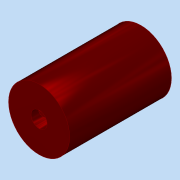
# Autodesk Inventor part: 3mm_.125inch_ShaftCoupler
Saved by Autodesk Inventor 2017.3 (Build 213256000, 256)
## iProperties
Created: 2018-07-04
Part Number: 3mm_.125inch_ShaftCoupler
Material: Aluminum 6061
Document SubType Name: Modeling
Designer: Derek Wider
Density: 2.7 g/cm^3
Appearance: Red Adonized
Author: Derek Wider
Autodesk Inventor part; units mm, degrees
ref_plane "YZ Plane" through (0, 0, 0) normal (1, 0, 0) x (0, 1, 0)
ref_plane "XZ Plane" through (0, 0, 0) normal (0, 1, 0) x (-1, 0, 0)
ref_plane "XY Plane" through (0, 0, 0) normal (0, 0, 1) x (1, 0, 0)
sketch "Sketch1" plane through (0, 0, 0) normal (0, 0, 1) x (1, 0, 0)
  circle A0 centre (0, 0) radius 6
  dimension "d0" = 12
  constraints: 1 centre point, 1 coincident
  measures "d0" diameter of A0
extrude "Extrusion1" add sketch "Sketch1" along normal blind 20
sketch "Sketch2" plane through (0, 0, 20) normal (0, 0, 1) x (1, 0, 0)
  circle A0 centre (0, 0) radius 1.585
  dimension "d3" = 3.17
  constraints: 1 centre point, 1 coincident
  measures "d3" diameter of A0
extrude "Extrusion2" cut sketch "Sketch2" against normal blind 10
sketch "Sketch3" plane through (0, 0, 0) normal (0, 0, -1) x (-1, 0, 0)
  circle A0 centre (0, 0) radius 1.5
  dimension "d6" = 3
  constraints: 1 centre point, 1 coincident
  measures "d6" diameter of A0
extrude "Extrusion3" cut sketch "Sketch3" against normal blind 10
sketch "Sketch4" plane through (0, 0, 0) normal (1, 0, 0) x (0, 1, 0)
  circle A0 centre (0, 17) radius 1.5
  circle A1 centre (0, 3) radius 1.5
  line L0 (6, 20) -> (-6, 20) projected
  point P0 (0, 0)
  dimension "d9" = 3
  dimension "d10" = 3
  dimension "d11" = 3
  constraints: 2 centre point, 1 equal radius
  measures "d9" diameter of A0
  measures "d10" distance of point (0, 0) A1.centre
  measures "d11" distance from line of L0 A0.centre
extrude "Extrusion4" cut sketch "Sketch4" against normal through all
equation "\"d11\" = d10"
body "Solid1"
